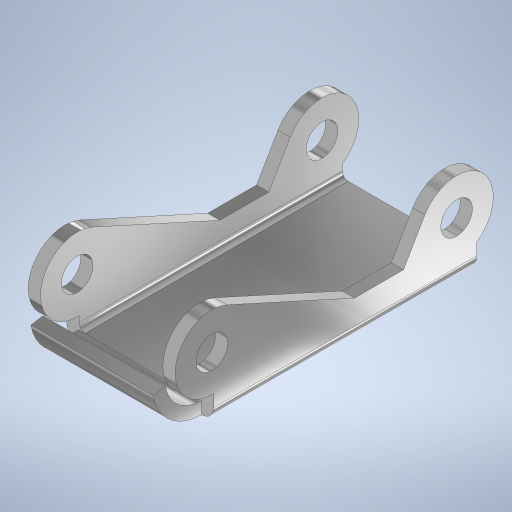
# Autodesk Inventor part: Linkage for 45 degree hinge
Saved by Autodesk Inventor 2024 (Build 280153000, 153)
## iProperties
Created: 2006-11-26
Part Number: Linkage for 45 degree hinge
Document SubType Name: Modeling
Designer: G.K.
Description: Linkage for 45 degree hinge
Authority: Design by UAB Čeli APS
Material: Steel
Mass: 3.96395 g
Surface Area: 11.4706 cm^2
Volume: 0.504962 cm^3
Density: 7.85 g/cm^3
Appearance: Chrome - Polished
Pavadinimas: Aselė
Šifras: L-90.00 002
Mase: 0.00396395
Autodesk Inventor part; units mm, degrees
ref_plane "YZ Plane" through (0, 0, 0) normal (1, 0, 0) x (0, 1, 0)
ref_plane "XZ Plane" through (0, 0, 0) normal (0, 1, 0) x (-1, 0, 0)
ref_plane "XY Plane" through (0, 0, 0) normal (0, 0, 1) x (1, 0, 0)
sketch "Sketch2" plane through (0, 0, 0) normal (1, 0, 0) x (0, 1, 0)
  line L0 (0, 10.4889) -> (0, -1.7482) projected
  line L1 (-17.7123, 0) -> (21.1316, 0) projected
  line L2 (13, 0) -> (13, 2)
  arc A0 (-7.4177, 7.7315) -> (-8.5, 2.0042) centre (-8.6583, 5) ccw
  line L3 (-8.5, 2.0042) -> (-8.5, 0)
  line L4 (7, 3) -> (8.7479, 6.0075)
  arc A1 (13, 2) -> (8.7479, 6.0075) centre (11.3417, 4.5) ccw
  circle A2 centre (11.3417, 4.5) radius 1.3
  circle A3 centre (-8.6583, 5) radius 1.3
  line L5 (7, 3) -> (3, 3)
  line L6 (3, 3) -> (-7.4177, 7.7315)
  dimension "d0" = 21.5
  dimension "d2" = 3
  dimension "d3" = 2
  dimension "d6" = 3
  dimension "d7" = 4.5
  dimension "d8" = 1.6583
  dimension "d9" = 5
  dimension "d10" = 20
  dimension "d16" = 3
  dimension "d17" = 2.6
  dimension "d30" = 13
  dimension "d31" = 4
  dimension "d32" = 6
  constraints: 10 end point, 4 centre point, 4 point on circle, 3 perpendicular, 2 coincident, 2 point on line, 2 tangent, 1 equal radius
  measures "d0" distance between parallel lines of L2 L3
  measures "d2" distance from line of L4.start L1
  measures "d3" distance from line of L2.end L1
  measures "d6" radius of A1
  measures "d7" distance from line of A1.centre L1
  measures "d8" distance from line of A1.centre L2
  measures "d9" distance from line of A0.centre L1
  measures "d10" horizontal distance of A0.centre A1.centre
  measures "d16" radius of A0
  measures "d17" diameter of A2
  measures "d30" distance between parallel lines of L0 L2
  measures "d31" distance of L4.start L5.end
  measures "d32" distance from line of L4.start L2
extrude "Extrusion1" add sketch "Sketch2" along normal mid plane 12
fillet "Fillet1" radius 1 2 edges at (6, 2.25, 0) (-6, 2.25, 0)
shell "Shell1" thickness 1 removed faces 9 at (2, -9.3053, 7.9294) at (2, 8.1653, 5.005) at (2, 13.3771, 2.2962) at (1.6667, -8.5, 1.3361) at (-1.6667, 13, 1.3333) at (2, 12.6249, 4.2915) at (2, -7.3751, 4.7915) at (-2, -3.9452, 6.1543) at (-2, 4.3333, 3)
sketch "Sketch4" plane through (0, 0, 0) normal (1, 0, 0) x (0, 1, 0)
  arc A0 (-11.4544, 3.4791) -> (-8.5, 1) centre (-8.5, 4) ccw
  arc A1 (-12.4392, 3.3054) -> (-8.5, 0) centre (-8.5, 4) ccw
  line L0 (-12.4392, 3.3054) -> (-11.4544, 3.4791)
  line L1 (-8.5, 1) -> (-8.5, 0)
  line L2 (-8.5, 0) -> (-8.5, 1) projected
  line L3 (-8.5, 0) -> (13, 0) projected
  line L4 (13, 1) -> (-8.5, 1) projected
  dimension "d40" = 3
  dimension "d42" = 1
  dimension "d43" = 80
  constraints: 5 point on circle, 4 end point, 3 point on line, 2 centre point, 1 tangent
  measures "d40" radius of A0
  measures "d42" distance of L0.start L0.end
  measures "d43" angle of L0 L1
extrude "Extrusion3" add sketch "Sketch4" along normal mid plane 10
fillet "Fillet2" radius 0.5 2 edges at (-5, 2.25, 1) (5, 2.25, 1)
body "Solid1"
